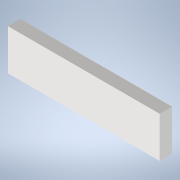
# Autodesk Inventor part: Part5
Saved by Autodesk Inventor 2022 (Build 260153000, 153)
## iProperties
Created: 2024-04-11
Part Number: Part5
Material: Generic
Document SubType Name: Modeling
Designer: Gotham City
Density: 1 g/cm^3
Appearance: Default
Author: Gotham City
Autodesk Inventor part; units mm, degrees
ref_plane "YZ Plane" through (0, 0, 0) normal (1, 0, 0) x (0, 1, 0)
ref_plane "XZ Plane" through (0, 0, 0) normal (0, 1, 0) x (-1, 0, 0)
ref_plane "XY Plane" through (0, 0, 0) normal (0, 0, 1) x (1, 0, 0)
sketch "Sketch1" plane through (0, 0, 0) normal (0, 0, 1) x (1, 0, 0)
  line L0 (0, 0) -> (27.85, 0)
  line L1 (27.85, 0) -> (27.85, -7.5)
  line L2 (27.85, -7.5) -> (0, -7.5)
  line L3 (0, -7.5) -> (0, 0)
  dimension "d0" = 27.85
  dimension "d1" = 7.5
  constraints: 8 end point, 2 parallel, 1 horizontal, 1 perpendicular
  measures "d0" distance of L1.end L2.end
  measures "d1" distance of L0.end L1.end
extrude "Extrusion1" add sketch "Sketch1" along normal blind 2.27
sketch "Sketch2" plane through (0, 0, 0) normal (0, 0, -1) x (-1, 0, 0)
  line L0 (-27.85, -7.5) -> (-27.85, 0) projected
  line L1 (-27.85, -3.75) -> (0, -3.75)
  line L2 (0, 0) -> (0, -7.5) projected
  point P0 (-13.925, -3.75)
  constraints: 3 midpoint, 2 end point
ref_plane "Work Plane1" through (27.85, -3.75, 0) normal (0, -1, 0) x (1, 0, 0)
ref_plane "Work Plane2" through (13.925, -3.75, 0) normal (-1, 0, 0) x (0, 0, 1)
body "Solid1"
